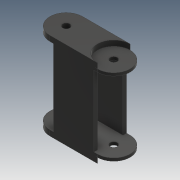
# Autodesk Inventor part: carrier-link
Saved by Autodesk Inventor 2017 (Build 210142000, 142)
## iProperties
Created: 2018-06-20
Part Number: carrier-link
Material: ABS Plastic
Document SubType Name: Modeling
Designer: Luiz Gustavo
Density: 1.06 g/cm^3
Appearance: Smooth - Black
Author: Luiz Gustavo
Autodesk Inventor part; units mm, degrees
ref_plane "YZ Plane" through (0, 0, 0) normal (1, 0, 0) x (0, 1, 0)
ref_plane "XZ Plane" through (0, 0, 0) normal (0, 1, 0) x (-1, 0, 0)
ref_plane "XY Plane" through (0, 0, 0) normal (0, 0, 1) x (1, 0, 0)
sketch "Sketch1" plane through (0, 0, 0) normal (0, 0, 1) x (1, 0, 0)
  arc A0 (0, 11.5) -> (0, -11.5) centre (0, 0) ccw
  line L0 (0, 0) -> (-33.5, 0) construction
  line L1 (-33.5, 11.5) -> (0, 11.5)
  line L2 (0, 11.5) -> (0, -11.5)
  line L3 (0, -11.5) -> (-33.5, -11.5)
  line L4 (-33.5, -11.5) -> (-33.5, 11.5)
  line L5 (-31, 9) -> (-2.5, 9)
  line L6 (-2.5, 9) -> (-2.5, -9)
  line L7 (-2.5, -9) -> (-31, -9)
  line L8 (-31, -9) -> (-31, 9)
  arc A1 (-33.5, -11.5) -> (-33.5, 11.5) centre (-33.5, 0) ccw
  arc A2 (-33.5, 11.5) -> (-33.5, -11.5) centre (-33.5, 0) ccw
  arc A3 (0, -11.5) -> (0, 11.5) centre (0, 0) ccw
  line L9 (-31, 9) -> (-31, 11.5)
  line L10 (-2.5, 9) -> (-2.5, 11.5)
  line L11 (-31, -9) -> (-31, -11.5)
  line L12 (-2.5, -9) -> (-2.5, -11.5)
  dimension "d0" = 2.5
  dimension "d1" = 2.5
  dimension "d2" = 2.5
  dimension "d3" = 2.5
  dimension "d4" = 18
  dimension "d5" = 33.5
  constraints: 26 end point, 8 point on circle, 4 centre point, 4 parallel, 4 perpendicular, 4 point on line, 3 horizontal, 2 coincident, 2 midpoint, 2 vertical, 1 equal radius
  measures "d0" distance between parallel lines of L1 L5
  measures "d1" distance between parallel lines of L3 L7
  measures "d2" distance between parallel lines of L4 L8
  measures "d3" distance between parallel lines of L6 L2
  measures "d4" distance of L5.end L6.end
  measures "d5" distance of L0.start L0.end
extrude "Extrusion3" add sketch "Sketch1" along normal mid plane 61.5 contours A0 L10 L1 | A0 L5 A1 L9 L1 L10 | L3 L12 A0 | A0 L7 A1 L5 | L9 A1 L1 | L12 L3 L11 A1 L7 A0 | A1 L7 L8 L5 | L5 L9 A1 | A1 L9 L8 L11 L4 | L4 A2 | L3 A1 L11 | A1 L11 L7
extrude "Extrusion4" add sketch "Sketch1" along normal mid plane 54 contours L2 A0 L12 L6 L10 | A3 L2 | L10 L5 A0 | L5 L6 L7 A0 | A0 L7 L12
extrude "Extrusion5" cut sketch "Sketch1" along normal mid plane 50
extrude "Extrusion7" cut sketch "Sketch1" along normal mid plane 54 contours L9 A1 L1 | A1 L7 L8 L5 | L5 L9 A1 | A1 L9 L8 L11 L4 | L4 A2 | L3 A1 L11 | A1 L11 L7
extrude "Extrusion6" add sketch "Sketch1" along normal mid plane 50 contours L10 L5 A0 | A0 L5 A1 L9 L1 L10 | L12 L3 L11 A1 L7 A0 | A0 L7 L12 | L5 L9 A1 | A1 L11 L7
hole "Hole1" at (-33.5, 0, 0) at (0, 0, 0) direction (0, 0, 1) diameter 5 end through all
hole "Hole2" at (0, 0, 0) at (-33.5, 0, 0) direction (0, 0, -1) diameter 5 end through all
equation "\"d1\" = d0"
equation "\"d2\" = d0"
equation "\"d3\" = d0"
body "Solid2"
